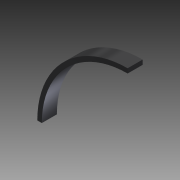
# Autodesk Inventor part: Rubber Cushion
Saved by Autodesk Inventor 2014 SP1 (Build 180222100, 222)
## iProperties
Created: 2013-03-21
Part Number: Rubber Cushion
Material: Rubber
Document SubType Name: Modeling
Designer: actoennies
Mass: 656.449 g
Surface Area: 987.571 cm^2
Volume: 705.859 cm^3
Density: 0.93 g/cm^3
Appearance: Rubber - Black - Version 1.1
Author: actoennies
Autodesk Inventor part; units mm, degrees
ref_plane "YZ Plane" through (0, 0, 0) normal (1, 0, 0) x (0, 1, 0)
ref_plane "XZ Plane" through (0, 0, 0) normal (0, 1, 0) x (-1, 0, 0)
ref_plane "XY Plane" through (0, 0, 0) normal (0, 0, 1) x (1, 0, 0)
sketch "Sketch1" plane through (0, 0, 0) normal (0, 0, 1) x (1, 0, 0)
  arc A0 (0, 381) -> (-381, 0) centre (0, 0) ccw
  arc A1 (0, 361.95) -> (-361.95, 0) centre (0, 0) ccw
  line L0 (0, 361.95) -> (0, 381)
  line L1 (-361.95, 0) -> (-381, 0)
  dimension "d0" = 762
  dimension "d1" = 19.05
  constraints: 4 end point, 4 point on circle, 2 centre point, 1 coincident, 1 perpendicular, 1 vertical
  measures "d0" diameter of A0
  measures "d1" radial gap between concentric circles of A0 A1
extrude "Extrusion1" add sketch "Sketch1" along normal blind 63.5
body "Solid1"
